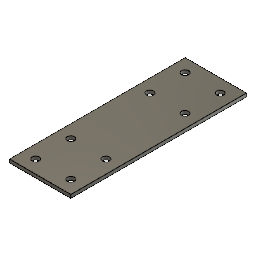
10part (Autodesk Fusion 360 design; units mm, degrees)
Autodesk Fusion 360 part; units mm, degrees
sketch "Sketch1" plane through (0, 0, 0) normal (0, 1, 0) x (1, 0, 0)
  line L0 (-17.5, 50) -> (17.5, 50)
  line L1 (17.5, 50) -> (17.5, -50)
  line L2 (17.5, -50) -> (-17.5, -50)
  line L3 (-17.5, -50) -> (-17.5, 50)
  circle A0 centre (-10, 42.5) radius 2
  circle A1 centre (10, 42.5) radius 2
  circle A2 centre (-10, 22.5) radius 2
  circle A3 centre (10, 22.5) radius 2
  line L4 (1.75, 0) -> (22.5, 0)
  circle A4 centre (-10, -42.5) radius 2
  circle A5 centre (10, -42.5) radius 2
  circle A6 centre (10, -22.5) radius 2
  circle A7 centre (-10, -22.5) radius 2
  dimension "d1" = 35
  dimension "d2" = 100
  dimension "d3" = 4
  dimension "d6" = 20
  dimension "d7" = -20
  dimension "d8" = 7.5
  dimension "d9" = 7.5
  constraint horizontal L0
  constraint vertical L1
  constraint horizontal L2
  constraint vertical L3
  constraint collinear origin L0.start L1.end
  constraint collinear origin L0.end L2.end
  constraint symmetric A0 L4 A4
  constraint symmetric A1 L4 A5
  constraint symmetric A2 L4 A7
  constraint symmetric A3 L4 A6
  measures "d1" distance of L0.start L0.end
  measures "d2" distance of L0.start L2.end
  measures "d3" diameter of A0
  measures "d8" distance of L3 A0.centre
  measures "d9" distance of L0 A0.centre
extrude "Extrude1" add sketch "Sketch1" along normal blind 2
equation "d9 = d8"
